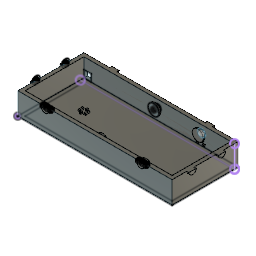
case bottom v2 (Autodesk Fusion 360 design; units mm, degrees)
Autodesk Fusion 360 part; units mm, degrees
note: some values were not read from the file. Set by a fixed rule: which sketch regions a step uses.
sketch "Sketch1" plane through (0, 0, 0) normal (0, 0, 1) x (1, 0, 0)
  line L0 (0, 90) -> (210, 90)
  line L1 (210, 90) -> (210, 0)
  line L2 (210, 0) -> (0, 0)
  line L3 (0, 0) -> (0, 90)
  line L4 (5, 5) -> (205, 5)
  line L5 (205, 5) -> (205, 85)
  line L6 (205, 85) -> (5, 85)
  line L7 (5, 85) -> (5, 5)
  dimension "d1" = 210
  dimension "d2" = 90
  dimension "d3" = 200
  dimension "d4" = 80
  dimension "d5" = 5
  dimension "d6" = 5
  constraint horizontal L0
  constraint vertical L1
  constraint horizontal L2
  constraint vertical L3
  constraint coincident L2.end L3
  constraint coincident L3.start L2
  constraint horizontal L4
  constraint vertical L5
  constraint horizontal L6
  constraint vertical L7
  measures "d1" distance of L0.start L0.end
  measures "d2" distance of L0.start L2.end
  measures "d3" distance of L4.start L4.end
  measures "d4" distance of L4.start L6.end
  measures "d5" distance of L3 L7
  measures "d6" distance of L2 L4
extrude "Extrude1" add sketch "Sketch1" along normal blind 5 contours L4 L5 L6 L7
extrude "Extrude2" add sketch "Sketch1" along normal blind 30
sketch "Sketch3" plane through (0, 85, 0) normal (0, -1, 0) x (1, 0, 0)
  line L0 (5, 5) -> (205, 5)
  line L1 (205, 5) -> (205, 30)
  line L2 (205, 30) -> (5, 30)
  line L3 (5, 30) -> (5, 5)
  circle A0 centre (105, 20) radius 5
  line L4 (210, 0) -> (210, 30)
  circle A1 centre (165, 20) radius 5
  dimension "d15" = 10
  dimension "d16" = 10
  dimension "d17" = 105
  dimension "d80" = 10
  dimension "d81" = 60
  measures "d15" diameter of A0
  measures "d16" distance of L2 A0.centre
  measures "d17" distance of A0.centre L4
  measures "d80" diameter of A1
  measures "d81" distance of A0.centre A1.centre
extrude "Extrude3" add sketch "Sketch3" along normal blind 5 contours A0
sketch "Sketch4" plane through (0, 80, 0) normal (0, -1, 0) x (1, 0, 0)
  circle A0 centre (105, 20) radius 5
  circle A1 centre (105, 20) radius 7.5
  dimension "d20" = 15
  constraint concentric A0 A1
  measures "d20" diameter of A1
extrude "Extrude4" add sketch "Sketch4" against normal blind 2
sketch "Sketch6" plane through (0, 85, 0) normal (0, -1, 0) x (1, 0, 0)
  circle A0 centre (105, 20) radius 5
  line L0 (5, 5) -> (205, 5)
  line L1 (205, 5) -> (205, 30)
  line L2 (205, 30) -> (5, 30)
  line L3 (5, 30) -> (5, 5)
  line L4 (162, 11) -> (168, 11)
  line L5 (168, 11) -> (168, 5)
  line L6 (168, 5) -> (162, 5)
  line L7 (162, 5) -> (162, 11)
  line L8 (5, 5) -> (205, 5)
  line L9 (210, 0) -> (210, 30)
  line L10 (162, 11) -> (168, 11)
  line L11 (168, 11) -> (168, 13)
  line L12 (168, 13) -> (162, 13)
  line L13 (162, 13) -> (162, 11)
  line L14 (168, 9) -> (170, 9)
  line L15 (170, 9) -> (170, 7)
  line L16 (170, 7) -> (168, 7)
  line L17 (168, 7) -> (168, 9)
  line L18 (162, 9) -> (160, 9)
  line L19 (160, 9) -> (160, 7)
  line L20 (160, 7) -> (162, 7)
  line L21 (162, 7) -> (162, 9)
  dimension "d91" = 6
  dimension "d92" = 6
  dimension "d93" = 42
  dimension "d94" = 2
  dimension "d95" = 2
  dimension "d96" = 2
  dimension "d97" = 2
  dimension "d98" = 2
  dimension "d99" = 2
  dimension "d100" = 2
  constraint horizontal L4
  constraint vertical L5
  constraint horizontal L6
  constraint vertical L7
  constraint collinear L6 L8
  constraint horizontal L10
  constraint vertical L11
  constraint horizontal L12
  constraint vertical L13
  constraint collinear L5 L11
  constraint horizontal L14
  constraint vertical L15
  constraint horizontal L16
  constraint vertical L17
  constraint coincident L5 L14.start
  constraint horizontal L18
  constraint vertical L19
  constraint horizontal L20
  constraint vertical L21
  constraint coincident L7 L18.start
  measures "d91" distance of L4.start L4.end
  measures "d92" distance of L4.start L6.end
  measures "d93" distance of L5 L9
  measures "d94" distance of L4.end L11.end
  measures "d95" distance of L14.start L14.end
  measures "d96" distance of L14.start L16.end
  measures "d97" distance of L10 L14
  measures "d98" distance of L18.start L18.end
  measures "d99" distance of L18.start L20.end
  measures "d100" distance of L8 L20
sketch "Sketch7" plane through (0, 0, 0) normal (-1, 0, 0) x (0, -1, 0)
  line L0 (-90, 0) -> (0, 0)
  line L1 (0, 0) -> (0, 30)
  line L2 (0, 30) -> (-90, 30)
  line L3 (-90, 30) -> (-90, 0)
  circle A0 centre (-25, 30) radius 5
  line L4 (-30, 30) -> (-20, 30)
  circle A1 centre (-65, 30) radius 5
  line L5 (-70, 30) -> (-60, 30)
  dimension "d31" = 10
  dimension "d32" = 10
  dimension "d47" = 25
  dimension "d48" = 25
  constraint coincident L4.start A0
  constraint coincident L4.end A0
  constraint coincident L5.start A1
  constraint coincident L5.end A1
  constraint coincident L2 A1.centre
  constraint coincident L2 A0.centre
  constraint horizontal L5
  constraint horizontal L4
  measures "d31" diameter of A0
  measures "d32" diameter of A1
  measures "d47" distance of L2.end A1.centre
  measures "d48" distance of L1 A0.centre
extrude "Extrude5" add sketch "Sketch7" along normal blind 3 contours L2 A1 L5 | L2 A0 L4 picked at (-66.5016, 29.2769) picked at (-23.5675, 28.3215)
ref_plane "WorkPlane1" through (0, 45, 0) normal (0, 1, 0) x (0, 0, 1)
mirror "Mirror1" about plane through (0, 45, 0) normal (0, 1, 0) of bodies 1 merged
ref_plane "WorkPlane2" through (105, 45, 15) normal (-1, 0, 0) x (0, -1, 0)
mirror "Mirror2" about plane through (105, 45, 15) normal (-1, 0, 0) of bodies 1 merged
sketch "Sketch8" plane through (0, 0, 0) normal (0, -1, 0) x (1, 0, 0)
  line L0 (0, 0) -> (210, 0)
  line L1 (210, 0) -> (210, 30)
  line L2 (210, 30) -> (0, 30)
  line L3 (0, 30) -> (0, 0)
  circle A0 centre (40, 30) radius 5
  circle A1 centre (170, 30) radius 5
  line L4 (35, 30) -> (45, 30)
  line L5 (165, 30) -> (175, 30)
  dimension "d39" = 10
  dimension "d40" = 10
  dimension "d41" = 40
  dimension "d42" = 40
  constraint coincident L2 A0.centre
  constraint coincident L2 A1.centre
  constraint coincident L2 L4.start
  constraint coincident A0 L4.start
  constraint coincident L2 L4.end
  constraint coincident A0 L4.end
  constraint coincident A1 L5.start
  constraint coincident L2 L5.start
  constraint coincident L2 L5.end
  constraint coincident A1 L5.end
  measures "d39" diameter of A1
  measures "d40" diameter of A0
  measures "d41" distance of L3 A0.centre
  measures "d42" distance of L1 A1.centre
extrude "Extrude6" add sketch "Sketch8" along normal blind 3 contours L2 A0 L4 | L2 A1 L5 picked at (38.7453, 27.2668) picked at (169.3911, 27.9517)
mirror "Mirror3" about plane through (0, 45, 0) normal (0, 1, 0) of bodies 1 merged
sketch "Sketch9" plane through (105, 85, 17.5) normal (0, -1, 0) x (1, 0, 0)
  line L0 (-100, -12.5) -> (-90, -12.5)
  line L1 (-90, -12.5) -> (-90, -2.5)
  line L2 (-90, -2.5) -> (-100, -2.5)
  line L3 (-100, -2.5) -> (-100, -12.5)
  line L4 (105, -17.5) -> (-105, -17.5)
  point P0 (-105, -17.5)
  dimension "d49" = 10
  dimension "d50" = 10
  dimension "d51" = 5
  dimension "d52" = 5
  constraint horizontal L0
  constraint vertical L1
  constraint horizontal L2
  constraint vertical L3
  measures "d49" distance of L0.start L0.end
  measures "d50" distance of L0.start L2.end
  measures "d51" distance of L0 L4
  measures "d52" distance of L3 P0
sketch "Sketch10" plane through (0, 0, 5) normal (0, 0, 1) x (-1, 0, 0)
  line L0 (-5, -85) -> (-5, -5)
  line L1 (-5, -5) -> (-205, -5)
  line L2 (-205, -5) -> (-205, -85)
  line L3 (-205, -85) -> (-5, -85)
  circle A0 centre (-45, -45) radius 20
  circle A1 centre (-105, -45) radius 20
  circle A2 centre (-165, -45) radius 20
  line L4 (-210, -90) -> (-210, 0)
  line L5 (-210, 0) -> (0, 0)
  line L6 (-42, -48) -> (-48, -48)
  line L7 (-48, -48) -> (-48, -42)
  line L8 (-48, -42) -> (-42, -42)
  line L9 (-42, -42) -> (-42, -48)
  line L10 (-48, -48) -> (-50, -48)
  line L11 (-50, -48) -> (-50, -42)
  line L12 (-50, -42) -> (-48, -42)
  line L13 (-48, -42) -> (-48, -48)
  line L14 (-42, -48) -> (-40, -48)
  line L15 (-40, -48) -> (-40, -42)
  line L16 (-40, -42) -> (-42, -42)
  line L17 (-42, -42) -> (-42, -48)
  line L18 (-44, -50) -> (-46, -50)
  line L19 (-46, -50) -> (-46, -48)
  line L20 (-46, -48) -> (-44, -48)
  line L21 (-44, -48) -> (-44, -50)
  line L22 (-44, -42) -> (-46, -42)
  line L23 (-46, -42) -> (-46, -40)
  line L24 (-46, -40) -> (-44, -40)
  line L25 (-44, -40) -> (-44, -42)
  dimension "d55" = 40
  dimension "d56" = 40
  dimension "d57" = 40
  dimension "d58" = 105
  dimension "d59" = 60
  dimension "d60" = 60
  dimension "d61" = 45
  dimension "d62" = 45
  dimension "d63" = 45
  dimension "d64" = 6
  dimension "d65" = 6
  dimension "d66" = 3
  dimension "d67" = 3
  dimension "d68" = 2
  dimension "d69" = 2
  dimension "d70" = 2
  dimension "d71" = 2
  dimension "d72" = 2
  dimension "d73" = 2
  dimension "d74" = 2
  dimension "d75" = 2
  dimension "d76" = 6
  constraint horizontal L6
  constraint vertical L7
  constraint horizontal L8
  constraint vertical L9
  constraint horizontal L10
  constraint vertical L11
  constraint horizontal L12
  constraint vertical L13
  constraint horizontal L14
  constraint vertical L15
  constraint horizontal L16
  constraint vertical L17
  constraint horizontal L18
  constraint vertical L19
  constraint horizontal L20
  constraint vertical L21
  constraint horizontal L22
  constraint vertical L23
  constraint horizontal L24
  constraint vertical L25
  constraint collinear L6 L20
  constraint collinear L8 L22
  constraint collinear L8 L16
  measures "d55" diameter of A0
  measures "d56" diameter of A1
  measures "d57" diameter of A2
  measures "d58" distance of A1.centre L4
  measures "d59" distance of A1.centre A2.centre
  measures "d60" distance of A0.centre A1.centre
  measures "d61" distance of A1.centre L5
  measures "d62" distance of A2.centre L5
  measures "d63" distance of A0.centre L5
  measures "d64" distance of L6.start L6.end
  measures "d65" distance of L6.start L8.end
  measures "d66" distance of A0.centre L6
  measures "d67" distance of A0.centre L9
  measures "d68" distance of L18.start L18.end
  measures "d69" distance of L18.start L20.end
  measures "d70" distance of L22.start L22.end
  measures "d71" distance of L22.start L24.end
  measures "d72" distance of L7 L23
  measures "d73" distance of L13 L19
  measures "d74" distance of L11.end L7.end
  measures "d75" distance of L15.end L8.end
  measures "d76" distance of L10.end L11.end
extrude "Extrude8" add sketch "Sketch10" along normal blind 2 contours L9 L14 L15 L16 L17 | L6 L18 L19 L20 L21 | L8 L22 L23 L24 L25 | L7 L10 L11 L12 L13
extrude "Extrude9" add sketch "Sketch3" along normal blind 5 contours A1
sketch "Sketch11" plane through (0, 80, 0) normal (0, -1, 0) x (1, 0, 0)
  circle A0 centre (165, 20) radius 5
  circle A1 centre (165, 20) radius 7.5
  dimension "d84" = 15
  constraint concentric A0 A1
  measures "d84" diameter of A1
extrude "Extrude10" add sketch "Sketch11" against normal blind 2
mirror "Mirror4" about plane through (0, 45, 0) normal (0, 1, 0) of bodies 1 merged
extrude "Extrude11" cut sketch "Sketch9" against normal blind 5
extrude "Extrude12" add sketch "Sketch6" along normal blind 2 contours L7 L18 L19 L20 L21 | L5 L14 L15 L16 L17 | L4 L10 L11 L12 L13
